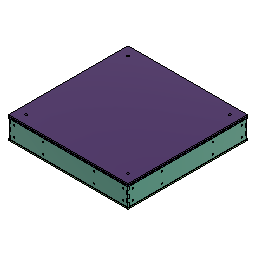
verbum-horologium (Autodesk Fusion 360 design; units mm, degrees)
Autodesk Fusion 360 part; units mm, degrees
note: some values were not read from the file. Chosen so that the rebuilt part matches the saved one: which bodies a step acts on. Set by a fixed rule: which sketch regions a step uses.
(part 1 of 5)
sketch "Sketch6" plane through (0, 0, 0) normal (0, 0, 1) x (1, 0, 0) in component "clock-face_black-polypropylene"
  line L0 (143.5, -143.5) -> (-143.5, -143.5)
  line L1 (-143.5, -143.5) -> (-143.5, 143.5)
  line L2 (-143.5, 143.5) -> (143.5, 143.5)
  line L3 (143.5, 143.5) -> (143.5, -143.5)
  line L4 (143.5, -143.5) -> (-143.5, 143.5) construction
  line L5 (-143.5, -143.5) -> (143.5, 143.5) construction
  line L6 (-143.5, -122.25) -> (143.5, -122.25) construction
  line L7 (-143.5, 0) -> (143.5, 0) construction
  circle A0 centre (-122.25, -122.25) radius 2.5
  circle A1 centre (122.25, -122.25) radius 2.5
  circle A2 centre (122.25, 122.25) radius 2.5
  circle A3 centre (-122.25, 122.25) radius 2.5
  line L8 (-143.5, 118.5) -> (143.5, 118.5) construction
  line L9 (0, 143.5) -> (0, -143.5) construction
  circle A4 centre (0, 118.5) radius 2.5
  line L10 (-93.5, 143.5) -> (-93.5, -143.5) construction
  line L11 (-143.5, 93.5) -> (143.5, 93.5) construction
  line L12 (-86, 86) -> (-101, 86)
  line L13 (-101, 86) -> (-101, 101)
  line L14 (-101, 101) -> (-86, 101)
  line L15 (-86, 101) -> (-86, 86)
  line L16 (-86, 86) -> (-101, 101) construction
  line L17 (-101, 86) -> (-86, 101) construction
  line L18 (-101, -101) -> (-101, -86)
  line L19 (-86, -86) -> (-86, -101)
  line L20 (-101, -86) -> (-86, -86)
  line L21 (-86, -101) -> (-101, -101)
  line L22 (101, -101) -> (86, -101)
  line L23 (86, -86) -> (101, -86)
  line L24 (86, -101) -> (86, -86)
  line L25 (101, -86) -> (101, -101)
  line L26 (101, 101) -> (101, 86)
  line L27 (86, 86) -> (86, 101)
  line L28 (101, 86) -> (86, 86)
  line L29 (86, 101) -> (101, 101)
  point P0 (-93.5, 93.5)
  dimension "d120" = 287
  dimension "d121" = 21.25
  dimension "d122" = 5
  dimension "d123" = 21.25
  dimension "d124" = 21.25
  dimension "d125" = 25
  dimension "d126" = 5
  dimension "d127" = 50
  dimension "d128" = 50
  dimension "d129" = 15
  dimension "d131" = 360
  constraint horizontal L0
  constraint perpendicular L0 L1
  constraint parallel L0 L2
  constraint parallel L1 L3
  constraint coincident L4 origin
  constraint coincident L5 origin
  constraint equal L1 L2
  constraint coincident L1 L6.start
  constraint coincident L3 L6.end
  constraint perpendicular L3 L6
  constraint midpoint L1 L7.start
  constraint midpoint L3 L7.end
  constraint coincident L6 A0.centre
  constraint coincident L6 A1.centre
  constraint equal A0 A1
  constraint symmetric L7 A0 A3
  constraint symmetric L7 A1 A2
  constraint coincident L1 L8.start
  constraint coincident L3 L8.end
  constraint perpendicular L3 L8
  constraint midpoint L2 L9.start
  constraint midpoint L0 L9.end
  constraint midpoint L8 A4.centre
  constraint coincident L2 L10.start
  constraint coincident L0 L10.end
  constraint perpendicular L0 L10
  constraint coincident L1 L11.start
  constraint coincident L3 L11.end
  constraint perpendicular L3 L11
  constraint horizontal L12
  constraint perpendicular L12 L13
  constraint parallel L12 L14
  constraint parallel L13 L15
  constraint coincident L16 P0
  constraint coincident L17 P0
  constraint coincident L10 P0
  constraint coincident L11 P0
  constraint equal L14 L15
  measures "d120" distance of L1.end L2.end
  measures "d121" distance of L0 L6
  measures "d122" diameter of A0
  measures "d123" distance of L1 A0.centre
  measures "d124" distance of L3 A1.centre
  measures "d125" distance of L2 L8
  measures "d126" diameter of A4
  measures "d127" distance of L2 L11
  measures "d128" distance of L1 L10
  measures "d129" distance of L13.end L14.end
extrude "Extrude3" add sketch "Sketch6" along normal blind 1.4 makes body 1 in component "clock-face_black-polypropylene"
sketch "Sketch1" plane through (0, 0, 1.4) normal (0, 0, 1) x (-1, 0, 0) in component "cover_clear-acrylic"
  line L0 (86, 86) -> (86, 101)
  line L1 (86, 101) -> (101, 101)
  line L2 (101, 101) -> (101, 86)
  line L3 (101, 86) -> (86, 86)
  circle A0 centre (-122.25, 122.25) radius 2.5
  line L4 (-86, 86) -> (-101, 86)
  line L5 (-101, 86) -> (-101, 101)
  line L6 (-101, 101) -> (-86, 101)
  line L7 (-86, 101) -> (-86, 86)
  line L8 (-86, -86) -> (-86, -101)
  line L9 (-86, -101) -> (-101, -101)
  line L10 (-101, -101) -> (-101, -86)
  line L11 (-101, -86) -> (-86, -86)
  circle A1 centre (0, -118.5) radius 2.5
  circle A2 centre (-122.25, -122.25) radius 2.5
  circle A3 centre (122.25, -122.25) radius 2.5
  circle A4 centre (122.25, 122.25) radius 2.5
  line L12 (101, -101) -> (86, -101)
  line L13 (86, -101) -> (86, -86)
  line L14 (86, -86) -> (101, -86)
  line L15 (101, -86) -> (101, -101)
  line L16 (-143.5, -143.5) -> (143.5, -143.5)
  line L17 (143.5, -143.5) -> (143.5, 143.5)
  line L18 (143.5, 143.5) -> (-143.5, 143.5)
  line L19 (-143.5, 143.5) -> (-143.5, -143.5)
  circle A5 centre (-122.25, -122.25) radius 2.5
  circle A6 centre (122.25, -122.25) radius 2.5
  line L20 (-143.5, -143.5) -> (143.5, -143.5)
  line L21 (-143.5, 143.5) -> (-143.5, -143.5)
  circle A7 centre (-122.25, 122.25) radius 2.5
  line L22 (143.5, 143.5) -> (-143.5, 143.5)
  circle A8 centre (122.25, 122.25) radius 2.5
  line L23 (143.5, -143.5) -> (143.5, 143.5)
extrude "Extrude1" add sketch "Sketch1" along normal blind 3 separate body contours L0 L1 L2 L3 | L4 L5 L6 L7 | L8 L9 L10 L11 | A1 | L12 L13 L14 L15 | L16 L17 L18 L19 L20 L21 L22 L23 picked at (91, 96) picked at (-91, 91) picked at (-96, -91) picked at (-0.062275, -117.668997) picked at (96, -96) picked at (0, 18.666667) makes body 2 in component "cover_clear-acrylic"
sketch "Sketch2" plane through (0, 0, 0) normal (0, 0, -1) x (1, 0, 0) in component "diffusion_white-acrylic"
  line L0 (-86, 101) -> (-86, 86)
  line L1 (-86, 86) -> (-101, 86)
  line L2 (-101, 86) -> (-101, 101)
  line L3 (-101, 101) -> (-86, 101)
  circle A0 centre (122.25, 122.25) radius 2.5
  line L4 (101, 86) -> (86, 86)
  line L5 (86, 86) -> (86, 101)
  line L6 (86, 101) -> (101, 101)
  line L7 (101, 101) -> (101, 86)
  line L8 (86, -101) -> (86, -86)
  line L9 (86, -86) -> (101, -86)
  line L10 (101, -86) -> (101, -101)
  line L11 (101, -101) -> (86, -101)
  circle A1 centre (0, -118.5) radius 2.5
  circle A2 centre (122.25, -122.25) radius 2.5
  circle A3 centre (-122.25, -122.25) radius 2.5
  circle A4 centre (-122.25, 122.25) radius 2.5
  line L12 (-86, -101) -> (-101, -101)
  line L13 (-101, -101) -> (-101, -86)
  line L14 (-101, -86) -> (-86, -86)
  line L15 (-86, -86) -> (-86, -101)
  line L16 (-143.5, -143.5) -> (143.5, -143.5)
  line L17 (143.5, -143.5) -> (143.5, 143.5)
  line L18 (143.5, 143.5) -> (-143.5, 143.5)
  line L19 (-143.5, 143.5) -> (-143.5, -143.5)
extrude "Extrude1'" add sketch "Sketch2" along normal blind 3 separate body contours L0 L1 L2 L3 | L4 L5 L6 L7 | L8 L9 L10 L11 | L12 L13 L14 L15 | L16 L17 L18 L19 picked at (-96, 96) picked at (96, 91) picked at (91, -91) picked at (-91, -96) picked at (0, 18.666667) makes body 3 in component "diffusion_white-acrylic"
sketch "Sketch3" plane through (0, 0, -3) normal (0, 0, -1) x (1, 0, 0) in component "spacer"
  circle A0 centre (-122.25, 122.25) radius 2.5
  circle A1 centre (122.25, -122.25) radius 2.5
  circle A2 centre (-122.25, -122.25) radius 2.5
  circle A3 centre (0, -118.5) radius 2.5
  circle A4 centre (122.25, 122.25) radius 2.5
  line L0 (-143.5, 143.5) -> (-143.5, -143.5)
  line L1 (-143.5, -143.5) -> (143.5, -143.5)
  line L2 (143.5, -143.5) -> (143.5, 143.5)
  line L3 (143.5, 143.5) -> (-143.5, 143.5)
  line L4 (-86, 101) -> (-86, 86)
  line L5 (-86, 86) -> (-101, 86)
  line L6 (-101, 86) -> (-101, 101)
  line L7 (-101, 101) -> (-86, 101)
  circle A5 centre (122.25, 122.25) radius 2.5
  line L8 (101, 86) -> (86, 86)
  line L9 (86, 86) -> (86, 101)
  line L10 (86, 101) -> (101, 101)
  line L11 (101, 101) -> (101, 86)
  line L12 (86, -101) -> (86, -86)
  line L13 (86, -86) -> (101, -86)
  line L14 (101, -86) -> (101, -101)
  line L15 (101, -101) -> (86, -101)
  circle A6 centre (0, -118.5) radius 2.5
  circle A7 centre (122.25, -122.25) radius 2.5
  circle A8 centre (-122.25, -122.25) radius 2.5
  circle A9 centre (-122.25, 122.25) radius 2.5
  line L16 (-86, -101) -> (-101, -101)
  line L17 (-101, -101) -> (-101, -86)
  line L18 (-101, -86) -> (-86, -86)
  line L19 (-86, -86) -> (-86, -101)
  line L20 (-143.5, -143.5) -> (143.5, -143.5)
  line L21 (143.5, -143.5) -> (143.5, 143.5)
  line L22 (143.5, 143.5) -> (-143.5, 143.5)
  line L23 (-143.5, 143.5) -> (-143.5, -143.5)
  line L24 (143.5, -143.5) -> (101, -101)
  line L25 (-143.5, -143.5) -> (-101, -101)
  line L26 (84, -101) -> (69, -101)
  line L27 (67, -101) -> (52, -101)
  line L28 (50, -101) -> (35, -101)
  line L29 (33, -101) -> (18, -101)
  line L30 (16, -101) -> (1, -101)
  line L31 (-1, -101) -> (-16, -101)
  line L32 (-18, -101) -> (-33, -101)
  line L33 (-35, -101) -> (-50, -101)
  line L34 (-52, -101) -> (-67, -101)
  line L35 (-69, -101) -> (-84, -101)
  line L36 (86, -101) -> (86, -108.5)
  line L37 (84, -101) -> (84, -108.5)
  line L38 (84, -108.5) -> (86, -108.5)
  line L39 (67, -101) -> (67, -108.5)
  line L40 (69, -101) -> (69, -108.5)
  line L41 (67, -108.5) -> (69, -108.5)
  line L42 (50, -101) -> (50, -108.5)
  line L43 (52, -101) -> (52, -108.5)
  line L44 (50, -108.5) -> (52, -108.5)
  line L45 (33, -101) -> (33, -108.5)
  line L46 (35, -101) -> (35, -108.5)
  line L47 (33, -108.5) -> (35, -108.5)
  line L48 (16, -101) -> (16, -108.5)
  line L49 (18, -101) -> (18, -108.5)
  line L50 (16, -108.5) -> (18, -108.5)
  line L51 (-1, -101) -> (-1, -108.5)
  line L52 (1, -101) -> (1, -108.5)
  line L53 (-1, -108.5) -> (1, -108.5)
  line L54 (-18, -101) -> (-18, -108.5)
  line L55 (-16, -101) -> (-16, -108.5)
  line L56 (-18, -108.5) -> (-16, -108.5)
  line L57 (-35, -101) -> (-35, -108.5)
  line L58 (-33, -101) -> (-33, -108.5)
  line L59 (-35, -108.5) -> (-33, -108.5)
  line L60 (-52, -101) -> (-52, -108.5)
  line L61 (-50, -101) -> (-50, -108.5)
  line L62 (-52, -108.5) -> (-50, -108.5)
  line L63 (-69, -101) -> (-69, -108.5)
  line L64 (-67, -101) -> (-67, -108.5)
  line L65 (-69, -108.5) -> (-67, -108.5)
  line L66 (-86, -101) -> (-86, -108.5)
  line L67 (-84, -101) -> (-84, -108.5)
  line L68 (-86, -108.5) -> (-84, -108.5)
  line L69 (122.25, -129.75) -> (-122.25, -129.75)
  circle A10 centre (122.25, -122.25) radius 7.5
  circle A11 centre (-122.25, -122.25) radius 7.5
  circle A12 centre (-122.25, -122.25) radius 8
  circle A13 centre (0, -118.5) radius 7.5
  circle A14 centre (-34, -118.5) radius 7.5
  circle A15 centre (-17, -118.5) radius 7.5
  circle A16 centre (17, -118.5) radius 7.5
  circle A17 centre (34, -118.5) radius 7.5
  circle A18 centre (122.25, -122.25) radius 8
  point P0 (107.25, -129.75)
  dimension "d158" = -17
  dimension "d159" = 0
  dimension "d160" = 7.5
  dimension "d161" = 5
  dimension "d162" = 15
  dimension "d163" = 0.5
  dimension "d164" = 15
  dimension "d167" = 15
  dimension "d170" = 17
  dimension "d171" = 0
  dimension "d174" = 0.5
  constraint coincident L1.end L2.start
  constraint coincident L14.end L15.start
  constraint coincident L0.end L1.start
  constraint coincident L16.end L17.start
  constraint coincident L12.start L15.end
  constraint perpendicular L15 L36
  constraint perpendicular L26 L37
  constraint perpendicular L36 L38
  constraint horizontal L69
  constraint concentric A1 A10
  constraint tangent L69 A10
  constraint coincident L69.start A10
  constraint concentric A8 A11
  constraint equal A10 A11
  constraint coincident L69.end A11
  constraint coincident L69 P0
  constraint concentric A3 A13
  measures "d160" distance of L12.start L36.end
  measures "d161" diameter of A1
  measures "d162" diameter of A10
  measures "d164" distance of L69.start P0
  measures "d167" diameter of A13
extrude "Extrude2" add sketch "Sketch3" along normal blind 7.5 separate body contours A1 A7 L24 A10 | A1 A7 L24 A10 | L24 L69 A10 A18 | L15 L16 L24 L25 L26 L27 L28 L29 L30 L31 L32 L33 L34 L35 L36 L37 L38 L39 L40 L41 L42 L43 L44 L45 L46 L47 L48 L49 L50 L51 L52 L53 L54 L55 L56 L57 L58 L59 L60 L61 L62 L63 L64 L65 L66 L67 L68 L69 A12 A18 picked at (126.798511, -118.622545) picked at (121.78987, -128.051035) picked at (119.52744, -129.402324) picked at (-74.834425, -119.783925) makes body 4 in component "spacer"
sketch "Sketch4" plane through (0, 0, -10.5) normal (0, 0, -1) x (1, 0, 0) in component "spacer"
  circle A0 centre (0, -118.5) radius 7.5
  circle A1 centre (122.25, -122.25) radius 2.5
  circle A2 centre (34, -118.5) radius 7.5
  circle A3 centre (17, -118.5) radius 7.5
  circle A4 centre (-17, -118.5) radius 7.5
  circle A5 centre (-34, -118.5) radius 7.5
  arc A6 (122.25, -129.75) -> (116.946699, -116.946699) centre (122.25, -122.25) ccw
  line L0 (116.946699, -116.946699) -> (101, -101)
  line L1 (101, -101) -> (86, -101)
  line L2 (86, -101) -> (86, -108.5)
  line L3 (86, -108.5) -> (84, -108.5)
  line L4 (84, -108.5) -> (84, -101)
  line L5 (84, -101) -> (69, -101)
  line L6 (69, -101) -> (69, -108.5)
  line L7 (69, -108.5) -> (67, -108.5)
  line L8 (67, -108.5) -> (67, -101)
  line L9 (67, -101) -> (52, -101)
  line L10 (52, -101) -> (52, -108.5)
  line L11 (52, -108.5) -> (50, -108.5)
  line L12 (50, -108.5) -> (50, -101)
  line L13 (50, -101) -> (35, -101)
  line L14 (35, -101) -> (35, -108.5)
  line L15 (35, -108.5) -> (33, -108.5)
  line L16 (33, -108.5) -> (33, -101)
  line L17 (33, -101) -> (18, -101)
  line L18 (18, -101) -> (18, -108.5)
  line L19 (18, -108.5) -> (16, -108.5)
  line L20 (16, -108.5) -> (16, -101)
  line L21 (16, -101) -> (1, -101)
  line L22 (1, -101) -> (1, -108.5)
  line L23 (1, -108.5) -> (-1, -108.5)
  line L24 (-1, -108.5) -> (-1, -101)
  line L25 (-1, -101) -> (-16, -101)
  line L26 (-16, -101) -> (-16, -108.5)
  line L27 (-16, -108.5) -> (-18, -108.5)
  line L28 (-18, -108.5) -> (-18, -101)
  line L29 (-18, -101) -> (-33, -101)
  line L30 (-33, -101) -> (-33, -108.5)
  line L31 (-33, -108.5) -> (-35, -108.5)
  line L32 (-35, -108.5) -> (-35, -101)
  line L33 (-35, -101) -> (-50, -101)
  line L34 (-50, -101) -> (-50, -108.5)
  line L35 (-50, -108.5) -> (-52, -108.5)
  line L36 (-52, -108.5) -> (-52, -101)
  line L37 (-52, -101) -> (-67, -101)
  line L38 (-67, -101) -> (-67, -108.5)
  line L39 (-67, -108.5) -> (-69, -108.5)
  line L40 (-69, -108.5) -> (-69, -101)
  line L41 (-69, -101) -> (-84, -101)
  line L42 (-84, -101) -> (-84, -108.5)
  line L43 (-84, -108.5) -> (-86, -108.5)
  line L44 (-86, -108.5) -> (-86, -101)
  line L45 (-86, -101) -> (-101, -101)
  line L46 (-101, -101) -> (-116.593146, -116.593146)
  arc A7 (-119.466118, -129.75) -> (-116.593146, -116.593146) centre (-122.25, -122.25) ccw
  line L47 (-119.466118, -129.75) -> (122.25, -129.75)
  line L48 (-143.5, -143.5) -> (-101, -101)
  circle A8 centre (-122.25, -122.25) radius 7.5
  line L49 (122.25, -129.75) -> (-122.25, -129.75)
  circle A9 centre (122.25, -122.25) radius 7.5
  circle A10 centre (-122.25, -122.25) radius 2.5
  circle A11 centre (122.25, -122.25) radius 8
extrude "Extrude3'" add sketch "Sketch4" along normal blind 7.5 contours L0 L1 L2 L3 L4 L5 L6 L7 L8 L9 L10 L11 L12 L13 L14 L15 L16 L17 L18 L19 L20 L21 L22 L23 L24 L25 L26 L27 L28 L29 L30 L31 L32 L33 L34 L35 L36 L37 L38 L39 L40 L41 L42 L43 L44 L45 L46 A7 L47 L48 L49 A11 | A7 L48 A8 L49 | L48 A8 A10 | L48 A8 A10 picked at (-74.782989, -119.717577) picked at (-114.615703, -122.797824) picked at (-121.812532, -128.053874) picked at (-126.69976, -125.997168) bodies 4 in component "spacer"
fillet "Fillet1" radius 1 6 edges at (116.593146, 116.593146, -14.25) (119.466118, 129.75, -14.25) (101, 101, -10.5) (-101, 101, -10.5) (-116.593146, 116.593146, -6.75) (-119.466118, 129.75, -6.75) on bodies 4 in component "spacer"
sketch "Sketch6 (2)" plane through (0, 0, -18) normal (0, 0, -1) x (1, 0, 0) in component "spacer"
  circle A0 centre (0, -118.5) radius 7.5
  circle A1 centre (34, -118.5) radius 7.5
  circle A2 centre (17, -118.5) radius 7.5
  circle A3 centre (-17, -118.5) radius 7.5
  circle A4 centre (-34, -118.5) radius 7.5
  circle A5 centre (-122.25, -122.25) radius 2.5
  arc A6 (-100.585786, -101) -> (-101.292893, -101.292893) centre (-100.585786, -102) ccw
  line L0 (-101.292893, -101.292893) -> (-116.946699, -116.946699)
  arc A7 (-116.946699, -116.946699) -> (-122.25, -129.75) centre (-122.25, -122.25) ccw
  line L1 (-122.25, -129.75) -> (116.02505, -129.75)
  arc A8 (116.02505, -129.75) -> (116.716711, -128.027778) centre (116.02505, -128.75) ccw
  arc A9 (115.999634, -117.256712) -> (116.716711, -128.027778) centre (122.25, -122.25) ccw
  arc A10 (115.999634, -117.256712) -> (115.925445, -115.925445) centre (115.218338, -116.632551) ccw
  line L2 (115.925445, -115.925445) -> (101.292893, -101.292893)
  arc A11 (101.292893, -101.292893) -> (100.585786, -101) centre (100.585786, -102) ccw
  line L3 (100.585786, -101) -> (86, -101)
  line L4 (86, -101) -> (86, -108.5)
  line L5 (86, -108.5) -> (84, -108.5)
  line L6 (84, -108.5) -> (84, -101)
  line L7 (84, -101) -> (69, -101)
  line L8 (69, -101) -> (69, -108.5)
  line L9 (69, -108.5) -> (67, -108.5)
  line L10 (67, -108.5) -> (67, -101)
  line L11 (67, -101) -> (52, -101)
  line L12 (52, -101) -> (52, -108.5)
  line L13 (52, -108.5) -> (50, -108.5)
  line L14 (50, -108.5) -> (50, -101)
  line L15 (50, -101) -> (35, -101)
  line L16 (35, -101) -> (35, -108.5)
  line L17 (35, -108.5) -> (33, -108.5)
  line L18 (33, -108.5) -> (33, -101)
  line L19 (33, -101) -> (18, -101)
  line L20 (18, -101) -> (18, -108.5)
  line L21 (18, -108.5) -> (16, -108.5)
  line L22 (16, -108.5) -> (16, -101)
  line L23 (16, -101) -> (1, -101)
  line L24 (1, -101) -> (1, -108.5)
  line L25 (1, -108.5) -> (-1, -108.5)
  line L26 (-1, -108.5) -> (-1, -101)
  line L27 (-1, -101) -> (-16, -101)
  line L28 (-16, -101) -> (-16, -108.5)
  line L29 (-16, -108.5) -> (-18, -108.5)
  line L30 (-18, -108.5) -> (-18, -101)
  line L31 (-18, -101) -> (-33, -101)
  line L32 (-33, -101) -> (-33, -108.5)
  line L33 (-33, -108.5) -> (-35, -108.5)
  line L34 (-35, -108.5) -> (-35, -101)
  line L35 (-35, -101) -> (-50, -101)
  line L36 (-50, -101) -> (-50, -108.5)
  line L37 (-50, -108.5) -> (-52, -108.5)
  line L38 (-52, -108.5) -> (-52, -101)
  line L39 (-52, -101) -> (-67, -101)
  line L40 (-67, -101) -> (-67, -108.5)
  line L41 (-67, -108.5) -> (-69, -108.5)
  line L42 (-69, -108.5) -> (-69, -101)
  line L43 (-69, -101) -> (-84, -101)
  line L44 (-84, -101) -> (-84, -108.5)
  line L45 (-84, -108.5) -> (-86, -108.5)
  line L46 (-86, -108.5) -> (-86, -101)
  line L47 (-86, -101) -> (-100.585786, -101)
  line L48 (-51, -112.5) -> (51, -112.5)
  line L49 (51, -112.5) -> (51, -124.5)
  line L50 (51, -124.5) -> (-51, -124.5)
  line L51 (-51, -124.5) -> (-51, -112.5)
  line L52 (-51, -112.5) -> (51, -124.5) construction
  line L53 (51, -112.5) -> (-51, -124.5) construction
  line L54 (86, -86) -> (86, -101)
  line L55 (101, -86) -> (86, -86)
  line L56 (101, -101) -> (101, -86)
  line L57 (100.585786, -101) -> (86, -101)
  line L58 (99.5, -101) -> (99.5, -110.5)
  line L59 (99.5, -110.5) -> (87.5, -110.5)
  line L60 (87.5, -110.5) -> (87.5, -101)
  line L61 (86, -101) -> (101, -86) construction
  line L62 (101, -101) -> (86, -86) construction
  line L63 (82.5, -101) -> (82.5, -110.5)
  line L64 (82.5, -110.5) -> (70.5, -110.5)
  line L65 (70.5, -110.5) -> (70.5, -101)
  line L66 (65.5, -101) -> (65.5, -110.5)
  line L67 (65.5, -110.5) -> (53.5, -110.5)
  line L68 (53.5, -110.5) -> (53.5, -101)
  line L69 (48.5, -101) -> (48.5, -110.5)
  line L70 (48.5, -110.5) -> (36.5, -110.5)
  line L71 (36.5, -110.5) -> (36.5, -101)
  line L72 (31.5, -101) -> (31.5, -110.5)
  line L73 (31.5, -110.5) -> (19.5, -110.5)
  line L74 (19.5, -110.5) -> (19.5, -101)
  line L75 (14.5, -101) -> (14.5, -110.5)
  line L76 (14.5, -110.5) -> (2.5, -110.5)
  line L77 (2.5, -110.5) -> (2.5, -101)
  line L78 (-2.5, -101) -> (-2.5, -110.5)
  line L79 (-2.5, -110.5) -> (-14.5, -110.5)
  line L80 (-14.5, -110.5) -> (-14.5, -101)
  line L81 (-19.5, -101) -> (-19.5, -110.5)
  line L82 (-19.5, -110.5) -> (-31.5, -110.5)
  line L83 (-31.5, -110.5) -> (-31.5, -101)
  line L84 (-36.5, -101) -> (-36.5, -110.5)
  line L85 (-36.5, -110.5) -> (-48.5, -110.5)
  line L86 (-48.5, -110.5) -> (-48.5, -101)
  line L87 (-53.5, -101) -> (-53.5, -110.5)
  line L88 (-53.5, -110.5) -> (-65.5, -110.5)
  line L89 (-65.5, -110.5) -> (-65.5, -101)
  line L90 (-70.5, -101) -> (-70.5, -110.5)
  line L91 (-70.5, -110.5) -> (-82.5, -110.5)
  line L92 (-82.5, -110.5) -> (-82.5, -101)
  line L93 (-87.5, -101) -> (-87.5, -110.5)
  line L94 (-87.5, -110.5) -> (-99.5, -110.5)
  line L95 (-99.5, -110.5) -> (-99.5, -101)
  point P0 (0, -118.5)
  point P1 (93.5, -110.5)
  point P2 (93.5, -93.5)
  dimension "d186" = 12
  dimension "d187" = 15
  dimension "d188" = 17
  dimension "d189" = 12
  dimension "d190" = 17
  dimension "d193" = -17
  dimension "d194" = 0
  constraint horizontal L48
  constraint perpendicular L48 L49
  constraint parallel L48 L50
  constraint parallel L49 L51
  constraint coincident L52 P0
  constraint coincident L53 P0
  constraint coincident P0 A0.centre
  constraint coincident L3 L58.start
  constraint perpendicular L57 L58
  constraint perpendicular L58 L59
  constraint coincident L3 L60.end
  constraint perpendicular L3 L60
  constraint midpoint L59 P1
  constraint coincident L3.end L4.start
  constraint coincident L55.start L56.end
  constraint coincident L56.start L62.start
  constraint coincident L54.start L55.end
  constraint midpoint L62 P2
  constraint vertical P1 P2
  measures "d186" distance of L48.end L49.end
  measures "d187" diameter of A4
  measures "d188" distance of A4.centre L51
  measures "d189" distance of L58.end L59.end
  measures "d190" distance of L59 P2
extrude "Extrude4" cut sketch "Sketch6 (2)" against normal blind 3 contours A0 A2 L48 L50 | A0 A3 L48 L50 | A1 A2 L48 L50 | A3 A4 L48 L50 | A1 L48 L49 L50 | A4 L48 L50 L51 | L47 L93 L94 L95 | L43 L90 L91 L92 | L3 L57 L58 L59 L60 | L39 L87 L88 L89 | L7 L63 L64 L65 | L35 L84 L85 L86 | L11 L66 L67 L68 | L31 L81 L82 L83 | L15 L69 L70 L71 | L27 L78 L79 L80 | L19 L72 L73 L74 | L23 L75 L76 L77 picked at (8.874809, -119.539288) picked at (-8.125191, -119.539288) picked at (25.874809, -119.539288) picked at (-25.125191, -119.539288) picked at (47.833333, -118.5) picked at (-47.826976, -118.678175) picked at (-91.5, -104.166667) picked at (-74.5, -104.166667) picked at (95.5, -104.166667) picked at (-57.5, -104.166667) picked at (78.5, -104.166667) picked at (-40.5, -104.166667) picked at (61.5, -104.166667) picked at (-23.5, -104.166667) picked at (44.5, -104.166667) picked at (-6.5, -104.166667) picked at (27.5, -104.166667) picked at (10.5, -104.166667) bodies 4 in component "spacer"
sketch "Sketch7" plane through (0, 0, -18) normal (0, 0, -1) x (1, 0, 0) in component "spacer"
  circle A0 centre (-122.25, -122.25) radius 2.5
  line L0 (12.5, -124.5) -> (4.5, -124.5)
  arc A1 (-4.5, -124.5) -> (4.5, -124.5) centre (0, -118.5) ccw
  line L1 (-4.5, -124.5) -> (-12.5, -124.5)
  arc A2 (-21.5, -124.5) -> (-12.5, -124.5) centre (-17, -118.5) ccw
  line L2 (-21.5, -124.5) -> (-29.5, -124.5)
  arc A3 (-38.5, -124.5) -> (-29.5, -124.5) centre (-34, -118.5) ccw
  line L3 (-38.5, -124.5) -> (-51, -124.5)
  line L4 (-51, -124.5) -> (-51, -112.5)
  line L5 (-51, -112.5) -> (-38.5, -112.5)
  arc A4 (-29.5, -112.5) -> (-38.5, -112.5) centre (-34, -118.5) ccw
  line L6 (-29.5, -112.5) -> (-21.5, -112.5)
  arc A5 (-12.5, -112.5) -> (-21.5, -112.5) centre (-17, -118.5) ccw
  line L7 (-12.5, -112.5) -> (-4.5, -112.5)
  arc A6 (4.5, -112.5) -> (-4.5, -112.5) centre (0, -118.5) ccw
  line L8 (4.5, -112.5) -> (12.5, -112.5)
  arc A7 (21.5, -112.5) -> (12.5, -112.5) centre (17, -118.5) ccw
  line L9 (21.5, -112.5) -> (29.5, -112.5)
  arc A8 (38.5, -112.5) -> (29.5, -112.5) centre (34, -118.5) ccw
  line L10 (38.5, -112.5) -> (51, -112.5)
  line L11 (51, -112.5) -> (51, -124.5)
  line L12 (51, -124.5) -> (38.5, -124.5)
  arc A9 (29.5, -124.5) -> (38.5, -124.5) centre (34, -118.5) ccw
  line L13 (29.5, -124.5) -> (21.5, -124.5)
  arc A10 (12.5, -124.5) -> (21.5, -124.5) centre (17, -118.5) ccw
  line L14 (86, -101) -> (86, -108.5)
  line L15 (86, -108.5) -> (84, -108.5)
  line L16 (84, -108.5) -> (84, -101)
  line L17 (84, -101) -> (82.5, -101)
  line L18 (82.5, -101) -> (82.5, -110.5)
  line L19 (82.5, -110.5) -> (70.5, -110.5)
  line L20 (70.5, -110.5) -> (70.5, -101)
  line L21 (70.5, -101) -> (69, -101)
  line L22 (69, -101) -> (69, -108.5)
  line L23 (69, -108.5) -> (67, -108.5)
  line L24 (67, -108.5) -> (67, -101)
  line L25 (67, -101) -> (65.5, -101)
  line L26 (65.5, -101) -> (65.5, -110.5)
  line L27 (65.5, -110.5) -> (53.5, -110.5)
  line L28 (53.5, -110.5) -> (53.5, -101)
  line L29 (53.5, -101) -> (52, -101)
  line L30 (52, -101) -> (52, -108.5)
  line L31 (52, -108.5) -> (50, -108.5)
  line L32 (50, -108.5) -> (50, -101)
  line L33 (50, -101) -> (48.5, -101)
  line L34 (48.5, -101) -> (48.5, -110.5)
  line L35 (48.5, -110.5) -> (36.5, -110.5)
  line L36 (36.5, -110.5) -> (36.5, -101)
  line L37 (36.5, -101) -> (35, -101)
  line L38 (35, -101) -> (35, -108.5)
  line L39 (35, -108.5) -> (33, -108.5)
  line L40 (33, -108.5) -> (33, -101)
  line L41 (33, -101) -> (31.5, -101)
  line L42 (31.5, -101) -> (31.5, -110.5)
  line L43 (31.5, -110.5) -> (19.5, -110.5)
  line L44 (19.5, -110.5) -> (19.5, -101)
  line L45 (19.5, -101) -> (18, -101)
  line L46 (18, -101) -> (18, -108.5)
  line L47 (18, -108.5) -> (16, -108.5)
  line L48 (16, -108.5) -> (16, -101)
  line L49 (16, -101) -> (14.5, -101)
  line L50 (14.5, -101) -> (14.5, -110.5)
  line L51 (14.5, -110.5) -> (2.5, -110.5)
  line L52 (2.5, -110.5) -> (2.5, -101)
  line L53 (2.5, -101) -> (1, -101)
  line L54 (1, -101) -> (1, -108.5)
  line L55 (1, -108.5) -> (-1, -108.5)
  line L56 (-1, -108.5) -> (-1, -101)
  line L57 (-1, -101) -> (-2.5, -101)
  line L58 (-2.5, -101) -> (-2.5, -110.5)
  line L59 (-2.5, -110.5) -> (-14.5, -110.5)
  line L60 (-14.5, -110.5) -> (-14.5, -101)
  line L61 (-14.5, -101) -> (-16, -101)
  line L62 (-16, -101) -> (-16, -108.5)
  line L63 (-16, -108.5) -> (-18, -108.5)
  line L64 (-18, -108.5) -> (-18, -101)
  line L65 (-18, -101) -> (-19.5, -101)
  line L66 (-19.5, -101) -> (-19.5, -110.5)
  line L67 (-19.5, -110.5) -> (-31.5, -110.5)
  line L68 (-31.5, -110.5) -> (-31.5, -101)
  line L69 (-31.5, -101) -> (-33, -101)
  line L70 (-33, -101) -> (-33, -108.5)
  line L71 (-33, -108.5) -> (-35, -108.5)
  line L72 (-35, -108.5) -> (-35, -101)
  line L73 (-35, -101) -> (-36.5, -101)
  line L74 (-36.5, -101) -> (-36.5, -110.5)
  line L75 (-36.5, -110.5) -> (-48.5, -110.5)
  line L76 (-48.5, -110.5) -> (-48.5, -101)
  line L77 (-48.5, -101) -> (-50, -101)
  line L78 (-50, -101) -> (-50, -108.5)
  line L79 (-50, -108.5) -> (-52, -108.5)
  line L80 (-52, -108.5) -> (-52, -101)
  line L81 (-52, -101) -> (-53.5, -101)
  line L82 (-53.5, -101) -> (-53.5, -110.5)
  line L83 (-53.5, -110.5) -> (-65.5, -110.5)
  line L84 (-65.5, -110.5) -> (-65.5, -101)
  line L85 (-65.5, -101) -> (-67, -101)
  line L86 (-67, -101) -> (-67, -108.5)
  line L87 (-67, -108.5) -> (-69, -108.5)
  line L88 (-69, -108.5) -> (-69, -101)
  line L89 (-69, -101) -> (-70.5, -101)
  line L90 (-70.5, -101) -> (-70.5, -110.5)
  line L91 (-70.5, -110.5) -> (-82.5, -110.5)
  line L92 (-82.5, -110.5) -> (-82.5, -101)
  line L93 (-82.5, -101) -> (-84, -101)
  line L94 (-84, -101) -> (-84, -108.5)
  line L95 (-84, -108.5) -> (-86, -108.5)
  line L96 (-86, -108.5) -> (-86, -101)
  line L97 (-86, -101) -> (-87.5, -101)
  line L98 (-87.5, -101) -> (-87.5, -110.5)
  line L99 (-87.5, -110.5) -> (-99.5, -110.5)
  line L100 (-99.5, -110.5) -> (-99.5, -101)
  line L101 (-99.5, -101) -> (-100.585786, -101)
  arc A11 (-100.585786, -101) -> (-101.292893, -101.292893) centre (-100.585786, -102) ccw
  line L102 (-101.292893, -101.292893) -> (-116.946699, -116.946699)
  arc A12 (-116.946699, -116.946699) -> (-122.25, -129.75) centre (-122.25, -122.25) ccw
  line L103 (-122.25, -129.75) -> (116.02505, -129.75)
  arc A13 (116.02505, -129.75) -> (116.716711, -128.027778) centre (116.02505, -128.75) ccw
  arc A14 (115.999634, -117.256712) -> (116.716711, -128.027778) centre (122.25, -122.25) ccw
  arc A15 (115.999634, -117.256712) -> (115.925445, -115.925445) centre (115.218338, -116.632551) ccw
  line L104 (115.925445, -115.925445) -> (101.292893, -101.292893)
  arc A16 (101.292893, -101.292893) -> (100.585786, -101) centre (100.585786, -102) ccw
  line L105 (100.585786, -101) -> (99.5, -101)
  line L106 (99.5, -101) -> (99.5, -110.5)
  line L107 (99.5, -110.5) -> (87.5, -110.5)
  line L108 (87.5, -110.5) -> (87.5, -101)
  line L109 (87.5, -101) -> (86, -101)
  circle A17 centre (61.125, -122.25) radius 7.5
  line L110 (68.625, -122.25) -> (53.625, -122.25) construction
  line L111 (53.625, -122.25) -> (53.625, -129.75)
  line L112 (53.625, -129.75) -> (68.625, -129.75)
  line L113 (68.625, -129.75) -> (68.625, -122.25)
  line L114 (0, -111) -> (0, -126) construction
  circle A18 centre (-61.125, -122.25) radius 7.5
  line L115 (-68.625, -129.75) -> (-68.625, -122.25)
  line L116 (-53.625, -122.25) -> (-53.625, -129.75)
  dimension "d214" = 244.5
  dimension "d215" = 15
  dimension "d216" = 61.125
  constraint tangent L103 A17
  constraint horizontal L110
  constraint vertical L111
  constraint horizontal L112
  constraint vertical L113
  constraint coincident L103 L111.end
  constraint coincident A17 L110.start
  constraint tangent A17 L113
  constraint coincident A17 L110.end
  constraint midpoint A6 L114.start
  constraint midpoint A1 L114.end
  constraint symmetric A17 L114 A18
  constraint symmetric L110.start L114 L115.end
  constraint symmetric L110.end L114 L116.start
  constraint symmetric L111.end L114 L116.end
  constraint symmetric L112.end L114 L115.start
  measures "d214" distance of A0.centre A14.centre
  measures "d215" diameter of A17
  measures "d216" distance of A14.centre A17.centre
extrude "Extrude5" cut sketch "Sketch7" against normal blind 11.25 contours L103 A17 L112 L113 | L103 A17 L111 L112 | A17 | L103 A18 L116 | L103 A18 L115 | A18 picked at (67.151526, -128.276526) picked at (55.098474, -128.276526) picked at (59.572883, -124.390368) picked at (-55.098474, -128.276526) picked at (-67.151526, -128.276526) picked at (-63.608101, -123.360086) bodies 4 in component "spacer"
fillet "Fillet2" radius 1 22 edges at (-86, 101, -10.5) (-84, 101, -10.5) (-69, 101, -10.5) (-67, 101, -10.5) (-52, 101, -10.5) (-50, 101, -10.5) (-35, 101, -10.5) (-33, 101, -10.5) (-18, 101, -10.5) (-16, 101, -10.5) (-1, 101, -10.5) (1, 101, -10.5) (16, 101, -10.5) (18, 101, -10.5) (33, 101, -10.5) (35, 101, -10.5) (50, 101, -10.5) (52, 101, -10.5) (67, 101, -10.5) (69, 101, -10.5) (84, 101, -10.5) (86, 101, -10.5) on bodies 4 in component "spacer"
fillet "Fillet2" radius 1 4 edges at (-68.625, 129.75, -12.375) (-53.625, 129.75, -12.375) (53.625, 129.75, -12.375) (68.625, 129.75, -12.375) on bodies 4 in component "spacer"
pattern_circular "C-Pattern1" count 4 over 360 about axis through (0, 0, 1.75) along (0, 0, 1) of bodies 4 makes body 5 at (-120.617099, 81.915963, -3) makes body 6 at (-81.915963, -120.617099, -3) makes body 7 at (120.617099, -81.915963, -3) in component "spacer"
sketch "Sketch2 (2)" plane through (0, 0, -18) normal (0, 0, -1) x (1, 0, 0) in component "led-pannel-frame_ply"
  circle A0 centre (-122.25, -122.25) radius 2.5 construction
  line L0 (12.5, -124.5) -> (4.5, -124.5) construction
  arc A1 (-4.5, -124.5) -> (4.5, -124.5) centre (0, -118.5) ccw construction
  line L1 (-4.5, -124.5) -> (-12.5, -124.5) construction
  arc A2 (-21.5, -124.5) -> (-12.5, -124.5) centre (-17, -118.5) ccw construction
  line L2 (-21.5, -124.5) -> (-29.5, -124.5) construction
  arc A3 (-38.5, -124.5) -> (-29.5, -124.5) centre (-34, -118.5) ccw construction
  line L3 (-38.5, -124.5) -> (-51, -124.5) construction
  line L4 (-51, -124.5) -> (-51, -112.5) construction
  line L5 (-51, -112.5) -> (-38.5, -112.5) construction
  arc A4 (-29.5, -112.5) -> (-38.5, -112.5) centre (-34, -118.5) ccw construction
  line L6 (-29.5, -112.5) -> (-21.5, -112.5) construction
  arc A5 (-12.5, -112.5) -> (-21.5, -112.5) centre (-17, -118.5) ccw construction
  line L7 (-12.5, -112.5) -> (-4.5, -112.5) construction
  arc A6 (4.5, -112.5) -> (-4.5, -112.5) centre (0, -118.5) ccw construction
  line L8 (4.5, -112.5) -> (12.5, -112.5) construction
  arc A7 (21.5, -112.5) -> (12.5, -112.5) centre (17, -118.5) ccw construction
  line L9 (21.5, -112.5) -> (29.5, -112.5) construction
  arc A8 (38.5, -112.5) -> (29.5, -112.5) centre (34, -118.5) ccw construction
  line L10 (38.5, -112.5) -> (51, -112.5) construction
  line L11 (51, -112.5) -> (51, -124.5) construction
  line L12 (51, -124.5) -> (38.5, -124.5) construction
  arc A9 (29.5, -124.5) -> (38.5, -124.5) centre (34, -118.5) ccw construction
  line L13 (29.5, -124.5) -> (21.5, -124.5) construction
  arc A10 (12.5, -124.5) -> (21.5, -124.5) centre (17, -118.5) ccw construction
  arc A11 (87, -101) -> (86, -102) centre (87, -102) ccw construction
  line L14 (86, -102) -> (86, -108.5) construction
  line L15 (86, -108.5) -> (84, -108.5) construction
  line L16 (84, -108.5) -> (84, -102) construction
  arc A12 (84, -102) -> (83, -101) centre (83, -102) ccw construction
  line L17 (83, -101) -> (82.5, -101) construction
  line L18 (82.5, -101) -> (82.5, -110.5) construction
  line L19 (82.5, -110.5) -> (70.5, -110.5) construction
  line L20 (70.5, -110.5) -> (70.5, -101) construction
  line L21 (70.5, -101) -> (70, -101) construction
  arc A13 (70, -101) -> (69, -102) centre (70, -102) ccw construction
  line L22 (69, -102) -> (69, -108.5) construction
  line L23 (69, -108.5) -> (67, -108.5) construction
  line L24 (67, -108.5) -> (67, -102) construction
  arc A14 (67, -102) -> (66, -101) centre (66, -102) ccw construction
  line L25 (66, -101) -> (65.5, -101) construction
  line L26 (65.5, -101) -> (65.5, -110.5) construction
  line L27 (65.5, -110.5) -> (53.5, -110.5) construction
  line L28 (53.5, -110.5) -> (53.5, -101) construction
  line L29 (53.5, -101) -> (53, -101) construction
  arc A15 (53, -101) -> (52, -102) centre (53, -102) ccw construction
  line L30 (52, -102) -> (52, -108.5) construction
  line L31 (52, -108.5) -> (50, -108.5) construction
  line L32 (50, -108.5) -> (50, -102) construction
  arc A16 (50, -102) -> (49, -101) centre (49, -102) ccw construction
  line L33 (49, -101) -> (48.5, -101) construction
  line L34 (48.5, -101) -> (48.5, -110.5) construction
  line L35 (48.5, -110.5) -> (36.5, -110.5) construction
  line L36 (36.5, -110.5) -> (36.5, -101) construction
  line L37 (36.5, -101) -> (36, -101) construction
  arc A17 (36, -101) -> (35, -102) centre (36, -102) ccw construction
  line L38 (35, -102) -> (35, -108.5) construction
  line L39 (35, -108.5) -> (33, -108.5) construction
  line L40 (33, -108.5) -> (33, -102) construction
  arc A18 (33, -102) -> (32, -101) centre (32, -102) ccw construction
  line L41 (32, -101) -> (31.5, -101) construction
  line L42 (31.5, -101) -> (31.5, -110.5) construction
  line L43 (31.5, -110.5) -> (19.5, -110.5) construction
  line L44 (19.5, -110.5) -> (19.5, -101) construction
  line L45 (19.5, -101) -> (19, -101) construction
  arc A19 (19, -101) -> (18, -102) centre (19, -102) ccw construction
  line L46 (18, -102) -> (18, -108.5) construction
  line L47 (18, -108.5) -> (16, -108.5) construction
  line L48 (16, -108.5) -> (16, -102) construction
  arc A20 (16, -102) -> (15, -101) centre (15, -102) ccw construction
  line L49 (15, -101) -> (14.5, -101) construction
  line L50 (14.5, -101) -> (14.5, -110.5) construction
  line L51 (14.5, -110.5) -> (2.5, -110.5) construction
  line L52 (2.5, -110.5) -> (2.5, -101) construction
  line L53 (2.5, -101) -> (2, -101) construction
  arc A21 (2, -101) -> (1, -102) centre (2, -102) ccw construction
  line L54 (1, -102) -> (1, -108.5) construction
  line L55 (1, -108.5) -> (-1, -108.5) construction
  line L56 (-1, -108.5) -> (-1, -102) construction
  arc A22 (-1, -102) -> (-2, -101) centre (-2, -102) ccw construction
  line L57 (-2, -101) -> (-2.5, -101) construction
  line L58 (-2.5, -101) -> (-2.5, -110.5) construction
  line L59 (-2.5, -110.5) -> (-14.5, -110.5) construction
  line L60 (-14.5, -110.5) -> (-14.5, -101) construction
  line L61 (-14.5, -101) -> (-15, -101) construction
  arc A23 (-15, -101) -> (-16, -102) centre (-15, -102) ccw construction
  line L62 (-16, -102) -> (-16, -108.5) construction
  line L63 (-16, -108.5) -> (-18, -108.5) construction
  line L64 (-18, -108.5) -> (-18, -102) construction
  arc A24 (-18, -102) -> (-19, -101) centre (-19, -102) ccw construction
  line L65 (-19, -101) -> (-19.5, -101) construction
  line L66 (-19.5, -101) -> (-19.5, -110.5) construction
  line L67 (-19.5, -110.5) -> (-31.5, -110.5) construction
  line L68 (-31.5, -110.5) -> (-31.5, -101) construction
  line L69 (-31.5, -101) -> (-32, -101) construction
  arc A25 (-32, -101) -> (-33, -102) centre (-32, -102) ccw construction
  line L70 (-33, -102) -> (-33, -108.5) construction
  line L71 (-33, -108.5) -> (-35, -108.5) construction
  line L72 (-35, -108.5) -> (-35, -102) construction
  arc A26 (-35, -102) -> (-36, -101) centre (-36, -102) ccw construction
  line L73 (-36, -101) -> (-36.5, -101) construction
  line L74 (-36.5, -101) -> (-36.5, -110.5) construction
  line L75 (-36.5, -110.5) -> (-48.5, -110.5) construction
  line L76 (-48.5, -110.5) -> (-48.5, -101) construction
  line L77 (-48.5, -101) -> (-49, -101) construction
  arc A27 (-49, -101) -> (-50, -102) centre (-49, -102) ccw construction
  line L78 (-50, -102) -> (-50, -108.5) construction
  line L79 (-50, -108.5) -> (-52, -108.5) construction
  line L80 (-52, -108.5) -> (-52, -102) construction
  arc A28 (-52, -102) -> (-53, -101) centre (-53, -102) ccw construction
  line L81 (-53, -101) -> (-53.5, -101) construction
  line L82 (-53.5, -101) -> (-53.5, -110.5) construction
  line L83 (-53.5, -110.5) -> (-65.5, -110.5) construction
  line L84 (-65.5, -110.5) -> (-65.5, -101) construction
  line L85 (-65.5, -101) -> (-66, -101) construction
  arc A29 (-66, -101) -> (-67, -102) centre (-66, -102) ccw construction
  line L86 (-67, -102) -> (-67, -108.5) construction
  line L87 (-67, -108.5) -> (-69, -108.5) construction
  line L88 (-69, -108.5) -> (-69, -102) construction
  arc A30 (-69, -102) -> (-70, -101) centre (-70, -102) ccw construction
  line L89 (-70, -101) -> (-70.5, -101) construction
  line L90 (-70.5, -101) -> (-70.5, -110.5) construction
  line L91 (-70.5, -110.5) -> (-82.5, -110.5) construction
  line L92 (-82.5, -110.5) -> (-82.5, -101) construction
  line L93 (-82.5, -101) -> (-83, -101) construction
  arc A31 (-83, -101) -> (-84, -102) centre (-83, -102) ccw construction
  line L94 (-84, -102) -> (-84, -108.5) construction
  line L95 (-84, -108.5) -> (-86, -108.5) construction
  line L96 (-86, -108.5) -> (-86, -102) construction
  arc A32 (-86, -102) -> (-87, -101) centre (-87, -102) ccw construction
  line L97 (-87, -101) -> (-87.5, -101) construction
  line L98 (-87.5, -101) -> (-87.5, -110.5) construction
  line L99 (-87.5, -110.5) -> (-99.5, -110.5) construction
  line L100 (-99.5, -110.5) -> (-99.5, -101) construction
  line L101 (-99.5, -101) -> (-100.585786, -101) construction
  arc A33 (-100.585786, -101) -> (-101.292893, -101.292893) centre (-100.585786, -102) ccw construction
  line L102 (-101.292893, -101.292893) -> (-116.946699, -116.946699) construction
  arc A34 (-116.946699, -116.946699) -> (-122.25, -129.75) centre (-122.25, -122.25) ccw construction
  line L103 (69.625, -129.75) -> (116.02505, -129.75) construction
  arc A35 (116.02505, -129.75) -> (116.716711, -128.027778) centre (116.02505, -128.75) ccw construction
  arc A36 (115.999634, -117.256712) -> (116.716711, -128.027778) centre (122.25, -122.25) ccw construction
  arc A37 (115.999634, -117.256712) -> (115.925445, -115.925445) centre (115.218338, -116.632551) ccw construction
  line L104 (115.925445, -115.925445) -> (101.292893, -101.292893) construction
  arc A38 (101.292893, -101.292893) -> (100.585786, -101) centre (100.585786, -102) ccw construction
  line L105 (100.585786, -101) -> (99.5, -101) construction
  line L106 (99.5, -101) -> (99.5, -110.5) construction
  line L107 (99.5, -110.5) -> (87.5, -110.5) construction
  line L108 (87.5, -110.5) -> (87.5, -101) construction
  line L109 (87.5, -101) -> (87, -101) construction
  arc A39 (116.946699, -116.946699) -> (129.75, -122.25) centre (122.25, -122.25) ccw construction
  line L110 (122.25, -129.75) -> (-122.25, -129.75)
  line L111 (-129.75, -122.25) -> (-129.75, 122.25)
  line L112 (-122.25, 129.75) -> (122.25, 129.75)
  line L113 (129.75, 122.25) -> (129.75, -122.25)
  line L114 (129.75, -129.75) -> (-129.75, 129.75) construction
  line L115 (-129.75, -129.75) -> (129.75, 129.75) construction
  arc A40 (122.25, -129.75) -> (129.75, -122.25) centre (122.25, -122.25) ccw
  arc A41 (-129.75, -122.25) -> (-122.25, -129.75) centre (-122.25, -122.25) ccw
  arc A42 (129.75, 122.25) -> (122.25, 129.75) centre (122.25, 122.25) ccw
  arc A43 (-122.25, 129.75) -> (-129.75, 122.25) centre (-122.25, 122.25) ccw
  circle A44 centre (122.25, -122.25) radius 2.5
  circle A45 centre (122.25, 122.25) radius 2.5
  circle A46 centre (-122.25, 122.25) radius 2.5
  circle A47 centre (-122.25, -122.25) radius 2.5
  line L116 (-101, -99.5) -> (-101, -87.5) construction
  line L117 (-101, -87.5) -> (-110.5, -87.5)
  line L118 (-110.5, -87.5) -> (-110.5, -99.5)
  line L119 (-110.5, -99.5) -> (-101, -99.5)
  line L120 (-105.75, -99.5) -> (-105.75, -87.5)
  line L121 (-51, -124.5) -> (-38.5, -124.5)
  arc A48 (-38.5, -112.5) -> (-38.5, -124.5) centre (-34, -118.5) ccw construction
  line L122 (-38.5, -112.5) -> (-51, -112.5)
  line L123 (-51, -112.5) -> (-51, -124.5)
  line L124 (-46.25, -124.5) -> (-46.25, -112.5)
  line L125 (-105.75, -82.5) -> (-105.75, -70.5)
  line L126 (-110.5, -70.5) -> (-110.5, -82.5)
  line L127 (-110.5, -82.5) -> (-101, -82.5)
  line L128 (-105.75, -65.5) -> (-105.75, -53.5)
  line L129 (-110.5, -53.5) -> (-110.5, -65.5)
  line L130 (-110.5, -65.5) -> (-101, -65.5)
  line L131 (-105.75, -48.5) -> (-105.75, -36.5)
  line L132 (-110.5, -36.5) -> (-110.5, -48.5)
  line L133 (-110.5, -48.5) -> (-101, -48.5)
  line L134 (-105.75, -31.5) -> (-105.75, -19.5)
  line L135 (-110.5, -19.5) -> (-110.5, -31.5)
  line L136 (-110.5, -31.5) -> (-101, -31.5)
  line L137 (-105.75, -14.5) -> (-105.75, -2.5)
  line L138 (-110.5, -2.5) -> (-110.5, -14.5)
  line L139 (-110.5, -14.5) -> (-101, -14.5)
  line L140 (-105.75, 2.5) -> (-105.75, 14.5)
  line L141 (-110.5, 14.5) -> (-110.5, 2.5)
  line L142 (-110.5, 2.5) -> (-101, 2.5)
  line L143 (-105.75, 19.5) -> (-105.75, 31.5)
  line L144 (-110.5, 31.5) -> (-110.5, 19.5)
  line L145 (-110.5, 19.5) -> (-101, 19.5)
  line L146 (-105.75, 36.5) -> (-105.75, 48.5)
  line L147 (-110.5, 48.5) -> (-110.5, 36.5)
  line L148 (-110.5, 36.5) -> (-101, 36.5)
  line L149 (-105.75, 53.5) -> (-105.75, 65.5)
  line L150 (-110.5, 65.5) -> (-110.5, 53.5)
  line L151 (-110.5, 53.5) -> (-101, 53.5)
  line L152 (-105.75, 70.5) -> (-105.75, 82.5)
  line L153 (-110.5, 82.5) -> (-110.5, 70.5)
  line L154 (-110.5, 70.5) -> (-101, 70.5)
  line L155 (-105.75, 87.5) -> (-105.75, 99.5)
  line L156 (-110.5, 99.5) -> (-110.5, 87.5)
  line L157 (-110.5, 87.5) -> (-101, 87.5)
  line L158 (-101, -70.5) -> (-110.5, -70.5)
  line L159 (-101, -53.5) -> (-110.5, -53.5)
  line L160 (-101, -36.5) -> (-110.5, -36.5)
  line L161 (-101, -19.5) -> (-110.5, -19.5)
  line L162 (-101, -2.5) -> (-110.5, -2.5)
  line L163 (-101, 14.5) -> (-110.5, 14.5)
  line L164 (-101, 31.5) -> (-110.5, 31.5)
  line L165 (-101, 48.5) -> (-110.5, 48.5)
  line L166 (-101, 65.5) -> (-110.5, 65.5)
  line L167 (-101, 82.5) -> (-110.5, 82.5)
  line L168 (-101, 99.5) -> (-110.5, 99.5)
  line L169 (0, -129.75) -> (0, 129.75) construction
  line L170 (110.5, -99.5) -> (101, -99.5)
  line L171 (105.75, -99.5) -> (105.75, -87.5)
  line L172 (110.5, -87.5) -> (110.5, -99.5)
  line L173 (101, -87.5) -> (110.5, -87.5)
  line L174 (110.5, -82.5) -> (101, -82.5)
  line L175 (110.5, -70.5) -> (110.5, -82.5)
  line L176 (105.75, -82.5) -> (105.75, -70.5)
  line L177 (101, -70.5) -> (110.5, -70.5)
  line L178 (110.5, -65.5) -> (101, -65.5)
  line L179 (110.5, -53.5) -> (110.5, -65.5)
  line L180 (105.75, -65.5) -> (105.75, -53.5)
  line L181 (101, -53.5) -> (110.5, -53.5)
  line L182 (110.5, -48.5) -> (101, -48.5)
  line L183 (110.5, -36.5) -> (110.5, -48.5)
  line L184 (105.75, -48.5) -> (105.75, -36.5)
  line L185 (101, -36.5) -> (110.5, -36.5)
  line L186 (110.5, -31.5) -> (101, -31.5)
  line L187 (110.5, -19.5) -> (110.5, -31.5)
  line L188 (105.75, -31.5) -> (105.75, -19.5)
  line L189 (101, -19.5) -> (110.5, -19.5)
  line L190 (110.5, -14.5) -> (101, -14.5)
  line L191 (105.75, -14.5) -> (105.75, -2.5)
  line L192 (110.5, -2.5) -> (110.5, -14.5)
  line L193 (101, -2.5) -> (110.5, -2.5)
  line L194 (110.5, 2.5) -> (101, 2.5)
  line L195 (110.5, 14.5) -> (110.5, 2.5)
  line L196 (105.75, 2.5) -> (105.75, 14.5)
  line L197 (101, 14.5) -> (110.5, 14.5)
  line L198 (110.5, 19.5) -> (101, 19.5)
  line L199 (105.75, 19.5) -> (105.75, 31.5)
  line L200 (110.5, 31.5) -> (110.5, 19.5)
  line L201 (101, 31.5) -> (110.5, 31.5)
  line L202 (110.5, 36.5) -> (101, 36.5)
  line L203 (110.5, 48.5) -> (110.5, 36.5)
  line L204 (105.75, 36.5) -> (105.75, 48.5)
  line L205 (101, 48.5) -> (110.5, 48.5)
  line L206 (110.5, 53.5) -> (101, 53.5)
  line L207 (110.5, 65.5) -> (110.5, 53.5)
  line L208 (105.75, 53.5) -> (105.75, 65.5)
  line L209 (101, 65.5) -> (110.5, 65.5)
  line L210 (110.5, 70.5) -> (101, 70.5)
  line L211 (110.5, 82.5) -> (110.5, 70.5)
  line L212 (105.75, 70.5) -> (105.75, 82.5)
  line L213 (101, 82.5) -> (110.5, 82.5)
  line L214 (110.5, 87.5) -> (101, 87.5)
  line L215 (105.75, 87.5) -> (105.75, 99.5)
  line L216 (110.5, 99.5) -> (110.5, 87.5)
  line L217 (101, 99.5) -> (110.5, 99.5)
  line L218 (46.25, -124.5) -> (46.25, -112.5)
  line L219 (51, -112.5) -> (51, -124.5)
  line L220 (38.5, -124.5) -> (51, -124.5)
  line L221 (51, -112.5) -> (38.5, -112.5)
  circle A49 centre (-34, 118.5) radius 7.5 construction
  circle A50 centre (-17, 118.5) radius 7.5 construction
  circle A51 centre (0, 118.5) radius 7.5
  circle A52 centre (17, 118.5) radius 7.5 construction
  circle A53 centre (34, 118.5) radius 7.5 construction
  arc A54 (68.625, -128.75) -> (69.625, -129.75) centre (69.625, -128.75) ccw
  line L222 (-122.25, -129.75) -> (-69.625, -129.75)
  arc A55 (-69.625, -129.75) -> (-68.625, -128.75) centre (-69.625, -128.75) ccw
  line L223 (-68.625, -128.75) -> (-68.625, -122.25)
  arc A56 (-53.625, -122.25) -> (-68.625, -122.25) centre (-61.125, -122.25) ccw
  line L224 (-53.625, -122.25) -> (-53.625, -128.75)
  arc A57 (-53.625, -128.75) -> (-52.625, -129.75) centre (-52.625, -128.75) ccw
  line L225 (-52.625, -129.75) -> (52.625, -129.75)
  arc A58 (52.625, -129.75) -> (53.625, -128.75) centre (52.625, -128.75) ccw
  line L226 (53.625, -128.75) -> (53.625, -122.25)
  arc A59 (68.625, -122.25) -> (53.625, -122.25) centre (61.125, -122.25) ccw
  line L227 (68.625, -122.25) -> (68.625, -128.75)
  circle A60 centre (-61.125, -122.25) radius 1.6
  circle A61 centre (61.125, -122.25) radius 1.6
  circle A62 centre (122.25, 61.125) radius 1.6
  circle A63 centre (122.25, -61.125) radius 1.6
  circle A64 centre (-61.125, 122.25) radius 1.6
  circle A65 centre (61.125, 122.25) radius 1.6
  circle A66 centre (-122.25, -61.125) radius 1.6
  circle A67 centre (-122.25, 61.125) radius 1.6
  circle A68 centre (-34, 123) radius 3 construction
  circle A69 centre (-34, 123) radius 1.6
  line L228 (-34, 118.5) -> (34, 118.5) construction
  circle A70 centre (-17, 123) radius 1.6
  circle A71 centre (0, 123) radius 1.6 construction
  circle A72 centre (17, 123) radius 1.6
  circle A73 centre (34, 123) radius 1.6
  circle A74 centre (-34, 114) radius 1.6
  circle A75 centre (-17, 114) radius 1.6
  circle A76 centre (17, 114) radius 1.6
  circle A77 centre (34, 114) radius 1.6
  dimension "d204" = 360
  dimension "d205" = 4.75
  dimension "d206" = 4.75
  dimension "d209" = 0
  dimension "d210" = 17
  dimension "d221" = 3.2
  dimension "d223" = 360
  dimension "d224" = 6
  dimension "d225" = 3.2
  dimension "d228" = 17
  dimension "d229" = 0
  constraint horizontal L110
  constraint perpendicular L110 L111
  constraint parallel L110 L112
  constraint parallel L111 L113
  constraint coincident L114 origin
  constraint coincident L115 origin
  constraint tangent A39 L110
  constraint tangent A39 L113
  constraint coincident L114.start L110
  constraint coincident L114.start L113
  constraint tangent L110 A40
  constraint tangent L113 A40
  constraint coincident A36.centre A39.centre
  constraint coincident L115.start L110
  constraint coincident L115.start L111
  constraint tangent L110 A41
  constraint tangent L111 A41
  constraint coincident A0.centre A34.centre
  constraint coincident L115.end L113
  constraint tangent L113 A42
  constraint tangent L112 A42
  constraint coincident L114.end L111
  constraint coincident L114.end L112
  constraint tangent L111 A43
  constraint tangent L112 A43
  constraint vertical A36.centre A42.centre
  constraint vertical A0.centre A43.centre